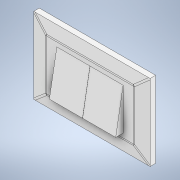
# Autodesk Inventor part: 스위치2
Saved by Autodesk Inventor 2022 (Build 260153000, 153)
## iProperties
Created: 2022-10-26
Part Number: 스위치2
Material: 일반
Document SubType Name: Modeling
Designer: whdls
Density: 1 g/cm^3
Appearance: 기본값
Author: whdls
Autodesk Inventor part; units mm, degrees
ref_plane "YZ Plane" through (0, 0, 0) normal (1, 0, 0) x (0, 1, 0)
sketch "스케치1" plane through (0, 0, 0) normal (0, 0, 1) x (1, 0, 0)
  line L0 (0, 0) -> (122, 0)
  line L1 (122, 0) -> (122, 80)
  line L2 (122, 80) -> (0, 80)
  line L3 (0, 80) -> (0, 0)
  dimension "d0" = 80
  dimension "d1" = 122
  constraints: 8 end point, 2 parallel, 1 horizontal, 1 perpendicular
  measures "d0" distance of L2.end L0.start
  measures "d1" distance of L1.end L2.end
extrude "돌출1" add sketch "스케치1" along normal blind 7.8
sketch "스케치2" plane through (0, 0, 7.8) normal (0, 0, 1) x (1, 0, 0)
  line L0 (26.25, 61.75) -> (95.75, 61.75)
  line L1 (95.75, 61.75) -> (95.75, 18.25)
  line L2 (95.75, 18.25) -> (26.25, 18.25)
  line L3 (26.25, 18.25) -> (26.25, 61.75)
  line L4 (0, 80) -> (0, 0) projected
  line L5 (0, 0) -> (122, 0) projected
  dimension "d4" = 43.5
  dimension "d5" = 69.5
  dimension "d6" = 26.25
  dimension "d7" = 18.25
  constraints: 8 end point, 2 parallel, 1 horizontal, 1 perpendicular
  measures "d4" distance of L2.end L0.start
  measures "d5" distance of L0.start L0.end
  measures "d6" distance between parallel lines of L4 L3
  measures "d7" distance between parallel lines of L5 L2
ref_plane "작업 평면1" through (95.75, 0, 0) normal (1, 0, 0) x (0, 0, -1)
sketch "스케치3" plane through (95.75, 0, 0) normal (1, 0, 0) x (0, 0, -1)
  line L0 (-7.8, 61.75) -> (-7.8, 18.25) projected
  line L1 (-7.8, 61.75) -> (-15.6034, 18.25)
  line L2 (-15.6034, 18.25) -> (-7.8, 18.25)
  point P0 (0, 0)
  dimension "d9" = 10.17
  constraints: 4 end point, 1 perpendicular
  measures "d9" angle of L0 L1
extrude "돌출2" add sketch "스케치3" against normal blind 34.7
ref_plane "작업 평면2" through (26.25, 0, 0) normal (-1, 0, 0) x (0, 0, 1)
sketch "스케치4" plane through (26.25, 0, 0) normal (-1, 0, 0) x (0, 0, 1)
  line L0 (7.8, 18.25) -> (7.8, 61.75) projected
  line L1 (7.8, 18.25) -> (15.6034, 18.25) projected
  line L2 (15.6034, 18.25) -> (7.8, 61.75) projected
  point P0 (0, 0)
extrude "돌출3" add sketch "스케치4" against normal blind 34.7
chamfer "모따기1" distance 15 distance2 2 1 edges at (122, 40, 7.8) measured on face at (61.0167, 73.9167, 7.8)
chamfer "모따기2" distance 15 distance2 2 1 edges at (0, 40, 7.8) measured on face at (8.75, 47.25, 7.8)
chamfer "모따기3" distance 13 distance2 2 1 edges at (61, 80, 7.8) measured on face at (61.0167, 73.9167, 7.8)
chamfer "모따기4" distance 13 distance2 2 1 edges at (61, 0, 7.8) measured on face at (60.9833, 6.0833, 7.8)
fillet "모깎기1" radius 10 8 edges at (114.5, 73.5, 6.8) (61, 67, 7.8) (107, 40, 7.8) (114.5, 6.5, 6.8) (61, 13, 7.8) (15, 40, 7.8) (7.5, 6.5, 6.8) (7.5, 73.5, 6.8)
